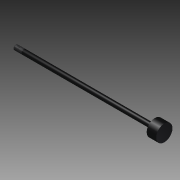
# Autodesk Inventor part: C-175-DPEE50_rod
Saved by Autodesk Inventor 2011 SP1 (Build 150282100, 282)
## iProperties
Created: 2016-10-01
Part Number: C-175-DPEE50_rod
Catalog Web Link: www.cadenas.de
Description: Standard Air Cylinder_rod-Original Line - Standard Air Cylinders
Vendor: BIMBA
Document SubType Name: Modeling
Designer: psAdmin
Manufacturer: BIMBA
Mass: 57.3445 g
Surface Area: 163.881 cm^2
Volume: 57.3445 cm^3
Density: 1 g/cm^3
Category: PARTsolutions
Company: BIMBA
Title: C-175-DPEE50_rod
Author: Cadenas PARTsolutions
Comments: Original Line - Standard Air Cylinders
PSOL_IDENT_0: {$CADENAS_DATA\23d-libs\bimba\bimba\bimba_imperial\bimba_full_line\original_line_cylinders\standard_
PSOL_IDENT_1: air_cylinders\rod.prj},298 {VTYP=3D},{NB=C-175-DPEE50_rod},{LINA=C-175-DPEE50_rod},{NN=Standard Air
PSOL_IDENT_2: Cylinder_rod},{DATE=22.09.2016 13:52:24},{GEOMDATE=10.09.2015 10:40:00},{VERSION=},{LINEID=80},{LINE
PSOL_IDENT_3: SUBID=-1},{WBVAR=STROKE,ACTING,MNT,DER,NR,BM,CO,M,EE,EEL,K,Q,Y,F,G,T,B,H,SER,SR,NT,W,E,HL,ST,STP,PRC
PSOL_IDENT_4: ,PB,COLOR1,FCD,RCD,BCD}  {NB=C-175-DPEE50_rod},{LINA=C-175-DPEE50_rod},{KT=DUMMY},{PN=C-175-DPEE5},{
PSOL_IDENT_5: DASH=-},{BORE=1.50000000},{BOREPN=17},{STROKE=5.000},{STROKEALG=[0.001:50/0.001]},{STROKE1=5.000},{A
PSOL_IDENT_6: CTING=D},{ACTINGALG= '' , 'Single Acting' , 'R' , 'Reverse Single Acting' , 'D' , 'Double Acting' },
PSOL_IDENT_7: {ACTINGPN=D},{MNT=P},{MNTALG= '' , 'Front Nose Mounting' , 'P' , 'Rear Pivot Mounting' , 'X' , 'Univ
PSOL_IDENT_8: ersal Pivot Mounting or Double End Mounting' , 'BF' , 'Front Block Mounting' , 'BR' , 'Rear Block Mo
PSOL_IDENT_9: unting for Vertical Positioning' , 'BFT' , 'Front Block Trunnion Mounting' , 'BRT' , 'Rear Block Tru
PSOL_IDENT_10: nnion Mounting' },{TYPE=C-},{MNTPN=P},{DER=},{DERALG= '' , 'N/A' },{NR=},{NRALG= '' , 'N/A' },{NRPN=
PSOL_IDENT_11: },{BM=},{BMALG= '' , 'N/A' },{BMPN=},{CO=},{COALG= '' , 'N/A' },{M=},{MALG= '', 'Without Magnet', 'M'
PSOL_IDENT_12: , 'With Magnet' },{EE=EE},{EEL=5},{EEMAX=7},{EEALG= '', 'Without Extra Extension', 'EE', 'With Extra
PSOL_IDENT_13: Extension' },{EELALG=[0.001:7/0.001]},{EEPN=EE5},{EEPN1=5.000},{K=},{KALG= '', 'Standard' , 'K' , '
PSOL_IDENT_14: Ports Rotated 90deg' },{KPN=},{Q=},{QALG= '' , 'Without Side Ported Rear Head' , 'Q' , 'With Side Po
PSOL_IDENT_15: rted Rear Head' },{QPN=},{Y=},{YALG= '' , 'Without Pivot Bushing' , 'Y' , 'With Pivot Bushing' },{YP
PSOL_IDENT_16: N=},{F=},{FALG= '', 'Standard', 'F', 'Molycoated Body' },{FPN=},{G=},{GPN=},{T=},{TALG= '' , 'Standa
PSOL_IDENT_17: rd' , 'N' , 'Low Temperature' , 'V' , 'High Temperature' },{NPN=},{VPN=},{B=},{BALG= '', 'Without Bu
PSOL_IDENT_18: mper' , 'B' , 'With Bumper' },{BPN=},{H=},{HALG= '', 'N/A' },{HPN=},{SER=},{SERALG= '' , 'Without Sp
PSOL_IDENT_19: ring Extend/Return' , 'JS' , 'With Spring Return' , 'JR' , 'With Spring Extend' },{SR=C},{SRALG= 'C'
PSOL_IDENT_20: , 'Carbon Steel Rod' , 'SR' , '303 Stainless Steel Rod' , '' , '303 Stainless Steel Rod1' },{SRPN=C
PSOL_IDENT_21: },{SRCON=1},{NT=},{NTPN=},{W=},{WALG= '' , 'Without Wiper' , 'W' , 'With Wiper' },{WPN=},{E=},{EALG=
PSOL_IDENT_22: '' , 'Without Special Lube and Seals' , 'E' , 'With Special Lube and Seals' },{EPN=},{HL=},{HLALG= ''
PSOL_IDENT_23: , 'Wihout Low Pressure Hydraulic' , 'HL' , 'With Low Pressure Hydraulic' },{ST=},{STALG= '' , 'With
PSOL_IDENT_24: out Switch Track' , 'T' , 'With Switch Track' },{STP=},{STPALG= '' , 'N/A' },{STPN=},{PRC=},{PRCALG=
PSOL_IDENT_25: '' , 'Without Piston Rod Clevis' , 'D-166-1' , 'With Piston Rod Clevis' },{PRCPN=},{PB=},{PBALG= ''
PSOL_IDENT_26: , 'Without Pivot Bracket' , 'D-167' , 'With Pivot Bracket' },{PBPN=},{TLEN=6.3025},{TEXT=0.433333},
PSOL_IDENT_27: {SPACE=0.247619},{FRAC=33.3800},{RGCON=},{RGDACCON=R},{RHCON=P},{RHCONON=1},{RHACCON=R},{FNUTCON=0},
PSOL_IDENT_28: {RNUTCON=0},{FNUTPN=},{RNUTPN=},{FNUTTRANS=0.0000},{RNUTTRANS=0.0000},{VHOLECON=0},{A1=1.8750},{A1N=
PSOL_IDENT_29: 1.3120},{A1P=1.8750},{A1B=2.3750},{A4=0.2525},{A4N=0.5000},{A4P=0.2525},{A5=0.0400},{A1H=1.75},{A1NH=
PSOL_IDENT_30: 0.6880},{A1PH=1.7500},{A1BH=1.3750},{A1SH=1.5000},{A2H=0.2500},{A2NH=0.2500},{LENGTH=4.3800},{LENGTH
PSOL_IDENT_31: 1=4.3800},{LENGTH2=4.4400},{MUL=5.0000},{MUL11=5.0000},{MUL22=13.4500},{MUL33=8.4500},{MUL2=5.0000},
PSOL_IDENT_32: {MUL211=5.0000},{MUL222=2.6900},{MUL233=1.6900},{SSS=10.0000},{RGLEN=1.6625},{RHLEN=1.1650},{SSS1=6.
PSOL_IDENT_33: 0000},{A13=1.3750},{THDLEN1=0.7500},{THD1=0.4375},{TAB=UNF},{THDLEN=0.7500},{THD=0.4375},{OD=1.5115}
PSOL_IDENT_34: ,{RODL=8.7550},{PL=0.8800},{RODDIA=0.4370},{HEX=0.4370},{RODTRANS=5.0000},{G1=0.0000},{ON=0},{G5=0.0
PSOL_IDENT_35: 000},{DERLEN=7.6250},{THOLE=0.2500},{WF=0.3800},{BADD=0.0000},{MADD=0.0000},{NVADD=0.000},{JRADD=0.0
PSOL_IDENT_36: 0000},{COLOR=0.00,0.00,0.00,0.00},{GROOVE=1},{HOL=0},{D7=0.3775},{H1=1.6160},{D1=1.5565},{D1RH=1.556
PSOL_IDENT_37: 5},{D1P=1.5800},{D1B=1.5565},{D1N=1.5565},{D1NRH=1.5565},{D1BRH=1.5800},{D1PRH=1.5565},{BOZO=0},{HAD
PSOL_IDENT_38: D=0.000},{COLOR1=0},{DEFL=0.0000},{HEXL=0.0000},{SSADD=0.0000},{WFL=0.2500},{MOVE=0.2500},{PRCL2=0.7
PSOL_IDENT_39: 5000},{PRCB=0.22000},{PRCTRANS=0.22000},{FCD=0},{RCD=0},{BCD=0}
NN: Standard Air Cylinder_rod
NT: Standard
NB: C-175-DPEE50_rod
NBSYN: $PN.$COLOR1._rod
LINA: C-175-DPEE50_rod
PN: C-175-DPEE5
BORE: 1.50000000
BOREPN: 17
STROKE: 5.000
ACTING: Double Acting
MNT: Rear Pivot Mounting
DER: N/A
NR: N/A
BM: N/A
CO: N/A
M: Without Magnet
EE: With Extra Extension
EEL: 5
K: Standard
Q: Without Side Ported Rear Head
Y: Without Pivot Bushing
F: Standard
G: Without Magnalube Lubrication
T: Standard
B: Without Bumper
H: N/A
SER: Without Spring Extend/Return
SR: Carbon Steel Rod
W: Without Wiper
E: Without Special Lube and Seals
HL: Wihout Low Pressure Hydraulic
ST: Without Switch Track
STP: N/A
PRC: Without Piston Rod Clevis
PB: Without Pivot Bracket
A1N: 1.3120
A1P: 1.8750
A1B: 2.3750
A4N: 0.5000
A4P: 0.2525
A5: 0.0400
A1NH: 0.6880
A1PH: 1.7500
A1BH: 1.3750
A1SH: 1.5000
A2NH: 0.2500
A13: 1.3750
THDLEN1: 0.7500
THD1: 0.4375
TAB: UNF
OD: 1.5115
RODDIA: 0.4370
HEX: 0.4370
G1: 0.0000
G5: 0.0000
THOLE: 0.2500
WF: 0.3800
GROOVE: 1
D7: 0.3775
D1P: 1.5800
D1B: 1.5565
D1N: 1.5565
D1NRH: 1.5565
D1BRH: 1.5800
D1PRH: 1.5565
COLOR1: 0
FCD: 0
RCD: 0
BCD: 0
SUPPLIER: BIMBA
ARTICLENO: C-175-DPEE50_rod
BOMINFO: C-175-DPEE50_rod
CREATOR: CADENAS GmbH
Autodesk Inventor part; units mm, degrees
ref_plane "YZ Plane" through (0, 0, 0) normal (1, 0, 0) x (0, 1, 0)
ref_plane "XZ Plane" through (0, 0, 0) normal (0, 1, 0) x (-1, 0, 0)
ref_plane "XY Plane" through (0, 0, 0) normal (0, 0, 1) x (1, 0, 0)
sketch "Sketch_1" plane through (0, 0, 0) normal (0, 0, 1) x (1, 0, 0)
  line L0 (323.977, 0) -> (-6.35, 0)
  line L1 (-6.35, 0) -> (-6.35, 5.5499)
  line L2 (-6.35, 5.5499) -> (301.625, 5.5499)
  line L3 (301.625, 5.5499) -> (301.625, 19.1453)
  line L4 (301.625, 19.1453) -> (323.977, 19.1453)
  line L5 (323.977, 19.1453) -> (323.977, 0)
  line L6 (323.977, 0) -> (-6.35, 0)
  constraints: 14 end point
revolve "Revolution1" add sketch "Sketch_1" angle 360 about axis through (323.977, 0, 0) along (1, 0, 0)
sketch "Sketch_3" plane through (0, 0, 0) normal (0, 0, 1) x (1, 0, 0)
  line L0 (-6.35, 0) -> (-25.4, 0)
  line L1 (-25.4, 0) -> (-25.4, 4.8006)
  line L2 (-25.4, 4.8006) -> (-24.6443, 5.5563)
  line L3 (-24.6443, 5.5563) -> (-6.35, 5.5563)
  line L4 (-6.35, 5.5563) -> (-6.35, 0)
  line L5 (-6.35, 0) -> (-25.4, 0)
  constraints: 12 end point
revolve "Revolution2" add sketch "Sketch_3" angle 360 about axis through (-6.35, 0, 0) along (1, 0, 0)
thread "Thread1" size "7/16-20 UNF" class "2A" standard "ANSI Unified Screw Threads" full length
sketch "Sketch_10" plane through (-6.35, 0, 0) normal (1, 0, 0) x (0, 0, -1)
  line L0 (-11.0998, -11.0998) -> (11.0998, -11.0998)
  line L1 (11.0998, -11.0998) -> (11.0998, 11.0998)
  line L2 (11.0998, 11.0998) -> (-11.0998, 11.0998)
  line L3 (-11.0998, 11.0998) -> (-11.0998, -11.0998)
  line L4 (-4.826, -5.5499) -> (4.826, -5.5499)
  line L5 (4.826, -5.5499) -> (4.826, 5.5499)
  line L6 (4.826, 5.5499) -> (-4.826, 5.5499)
  line L7 (-4.826, 5.5499) -> (-4.826, -5.5499)
  constraints: 16 end point
extrude "Extrusion1" cut sketch "Sketch_10" along normal blind 6.35
ref_plane "dia1_XY" through (-6.35, 5.5499, 0) normal (1, 0, 0) x (0, 0, -1)
ref_plane "dia1_YZ" through (-6.35, 5.5499, 0) normal (0, 0, -1) x (0, 1, 0)
ref_plane "dia1_ZX" through (-6.35, 5.5499, 0) normal (0, 1, 0) x (1, 0, 0)
ref_plane "dia12_XY" through (0, 0, 19.7675) normal (1, 0, 0) x (0, 0, -1)
ref_plane "dia12_YZ" through (0, 0, 19.7675) normal (0, 0, -1) x (0, 1, 0)
ref_plane "dia12_ZX" through (0, 0, 19.7675) normal (0, 1, 0) x (1, 0, 0)
ref_plane "dia2_XY" through (-6.35, -5.5499, 0) normal (1, 0, 0) x (0, 0, -1)
ref_plane "dia2_YZ" through (-6.35, -5.5499, 0) normal (0, 0, -1) x (0, 1, 0)
ref_plane "dia2_ZX" through (-6.35, -5.5499, 0) normal (0, 1, 0) x (1, 0, 0)
ref_plane "dia22_XY" through (0, 0, -19.7675) normal (1, 0, 0) x (0, 0, -1)
ref_plane "dia22_YZ" through (0, 0, -19.7675) normal (0, 0, -1) x (0, 1, 0)
ref_plane "dia22_ZX" through (0, 0, -19.7675) normal (0, 1, 0) x (1, 0, 0)
ref_plane "rl1_XY" through (-25.4, 0, 0) normal (1, 0, 0) x (0, 0, -1)
ref_plane "rl1_YZ" through (-25.4, 0, 0) normal (0, 0, -1) x (0, 1, 0)
ref_plane "rl1_ZX" through (-25.4, 0, 0) normal (0, 1, 0) x (1, 0, 0)
ref_plane "rl2_XY" through (-6.35, 0, 0) normal (1, 0, 0) x (0, 0, -1)
ref_plane "rl2_YZ" through (-6.35, 0, 0) normal (0, 0, -1) x (0, 1, 0)
ref_plane "rl2_ZX" through (-6.35, 0, 0) normal (0, 1, 0) x (1, 0, 0)
ref_plane "rod_cp_XY" through (0, 0, 0) normal (1, 0, 0) x (0, 0, -1)
ref_plane "rod_cp_YZ" through (0, 0, 0) normal (0, 0, -1) x (0, 1, 0)
ref_plane "rod_cp_ZX" through (0, 0, 0) normal (0, 1, 0) x (1, 0, 0)
ref_plane "thd1_XY" through (-25.4, 5.5563, 0) normal (1, 0, 0) x (0, 0, -1)
ref_plane "thd1_YZ" through (-25.4, 5.5563, 0) normal (0, 0, -1) x (0, 1, 0)
ref_plane "thd1_ZX" through (-25.4, 5.5563, 0) normal (0, 1, 0) x (1, 0, 0)
ref_plane "thd2_XY" through (-25.4, -5.5563, 0) normal (1, 0, 0) x (0, 0, -1)
ref_plane "thd2_YZ" through (-25.4, -5.5563, 0) normal (0, 0, -1) x (0, 1, 0)
ref_plane "thd2_ZX" through (-25.4, -5.5563, 0) normal (0, 1, 0) x (1, 0, 0)
ref_plane "to_rod_clevis_XY" through (-30.988, 0, 0) normal (1, 0, 0) x (0, 0, -1)
ref_plane "to_rod_clevis_YZ" through (-30.988, 0, 0) normal (0, 0, -1) x (0, 1, 0)
ref_plane "to_rod_clevis_ZX" through (-30.988, 0, 0) normal (0, 1, 0) x (1, 0, 0)
ref_plane "wf1_XY" through (-6.35, 0, 0) normal (1, 0, 0) x (0, 0, -1)
ref_plane "wf1_YZ" through (-6.35, 0, 0) normal (0, 0, -1) x (0, 1, 0)
ref_plane "wf1_ZX" through (-6.35, 0, 0) normal (0, 1, 0) x (1, 0, 0)
ref_plane "wf2_XY" through (0, 0, 0) normal (1, 0, 0) x (0, 0, -1)
ref_plane "wf2_YZ" through (0, 0, 0) normal (0, 0, -1) x (0, 1, 0)
ref_plane "wf2_ZX" through (0, 0, 0) normal (0, 1, 0) x (1, 0, 0)
ref_plane "wfw1_XY" through (-6.35, 0, -4.826) normal (0, 1, 0) x (1, 0, 0)
ref_plane "wfw1_YZ" through (-6.35, 0, -4.826) normal (1, 0, 0) x (0, 0, -1)
ref_plane "wfw1_ZX" through (-6.35, 0, -4.826) normal (0, 0, -1) x (0, 1, 0)
ref_plane "wfw2_XY" through (-6.35, 0, 4.826) normal (0, 1, 0) x (1, 0, 0)
ref_plane "wfw2_YZ" through (-6.35, 0, 4.826) normal (1, 0, 0) x (0, 0, -1)
ref_plane "wfw2_ZX" through (-6.35, 0, 4.826) normal (0, 0, -1) x (0, 1, 0)
body "Solid1"
